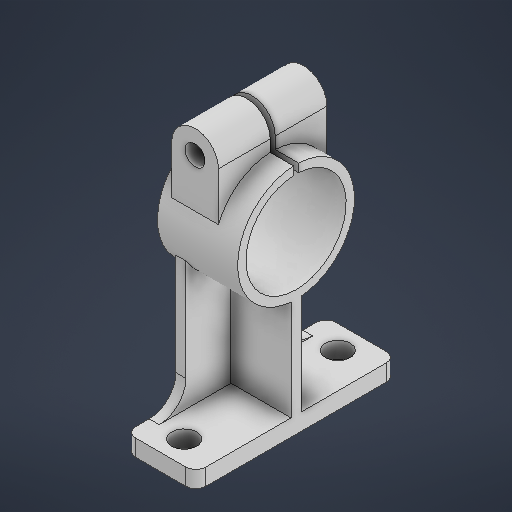
# Autodesk Inventor part: Pieza4
Saved by Autodesk Inventor 2026.1 (Build 301233020, 233B)
## iProperties
Created: 2026-02-14
Part Number: Pieza4
Material: Genérico
Document SubType Name: Modeling
Designer: UPN
Density: 1 g/cm^3
Appearance: Valor por defecto
Author: UPN
Autodesk Inventor part; units mm, degrees
note: some values were not read from the file. Chosen so that the rebuilt part matches the saved one: direction of "Hole1".
ref_plane "YZ Plane" through (0, 0, 0) normal (1, 0, 0) x (0, 1, 0)
ref_plane "XZ Plane" through (0, 0, 0) normal (0, 1, 0) x (-1, 0, 0)
sketch "Boceto1" plane through (0, 0, 0) normal (0, 1, 0) x (-1, 0, 0)
  line L0 (-15, 60) -> (15, 60)
  line L1 (21, 54) -> (21, -54)
  line L2 (15, -60) -> (-15, -60)
  line L3 (-21, -54) -> (-21, 54)
  line L4 (-21, 60) -> (21, -60) construction
  line L5 (21, 60) -> (-21, -60) construction
  arc A0 (21, 54) -> (15, 60) centre (15, 54) ccw
  arc A1 (-15, 60) -> (-21, 54) centre (-15, 54) ccw
  arc A2 (-21, -54) -> (-15, -60) centre (-15, -54) ccw
  arc A3 (15, -60) -> (21, -54) centre (15, -54) ccw
  circle A4 centre (0, 46) radius 7.5
  circle A5 centre (0, -46) radius 7.5
  point P0 (0, 0)
  dimension "d0" = 42
  dimension "d1" = 120
  dimension "d2" = 6
  dimension "d3" = 15
  dimension "d13" = 46
  dimension "d14" = 46
  constraints: 12 end point, 8 point on circle, 8 point on line, 8 tangent, 6 centre point, 4 equal radius, 2 midpoint, 2 parallel, 2 vertical alignment, 1 horizontal, 1 perpendicular
  measures "d0" distance of L4.end L5.end
  measures "d1" distance of L5.start L4.end
  measures "d2" radius of A0
  measures "d3" diameter of A4
  measures "d13" distance of A4.centre point (0, 0)
  measures "d14" distance of point (0, 0) A5.centre
extrude "Extrusión1" add sketch "Boceto1" along normal blind 10
sketch "Boceto2" plane through (-21, 0, -54) normal (-1, 0, 0) x (0, 0, 1)
  line L0 (0, 10) -> (108, 10) construction
  line L1 (24, 86.9722) -> (24, 26)
  line L2 (84, 86.9722) -> (84, 26)
  line L3 (0, 0) -> (108, 0) projected
  arc A0 (84, 26) -> (100, 10) centre (100, 26) ccw
  arc A1 (8, 10) -> (24, 26) centre (8, 26) ccw
  line L4 (92.5, 10) -> (107.5, 10) construction
  line L5 (0.5, 10) -> (15.5, 10) construction
  circle A2 centre (54, 105) radius 35
  line L6 (8, 10) -> (100, 10)
  point P0 (54, 0)
  point P1 (24, 10)
  point P2 (84, 10)
  point P3 (54, 0)
  point P4 (54, 0)
  point P5 (54, 10)
  dimension "d10" = 16
  dimension "d16" = 35
  dimension "d17" = 95
  constraints: 6 end point, 6 point on circle, 4 midpoint, 3 centre point, 3 vertical alignment, 2 point on line, 2 tangent, 2 vertical, 1 collinear, 1 equal radius, 6 other
  measures "d10" radius of A0
  measures "d16" radius of A2
  measures "d17" distance of A2.centre point (54, 10)
extrude "Extrusión2" add sketch "Boceto2" against normal blind 6 contours A2 L2 A0 L6 A1 L1
ref_plane "Plano de trabajo1" through (-18, 0, -54) normal (1, 0, 0) x (0, 0, -1)
sketch "Boceto3" plane through (-18, 0, -54) normal (1, 0, 0) x (0, 0, -1)
  arc A0 (-84, 86.9722) -> (-24, 86.9722) centre (-54, 105) ccw projected
  circle A1 centre (-54, 105) radius 35
  circle A2 centre (-54, 105) radius 30
  line L0 (-57, 10) -> (-51, 10)
  line L1 (-51, 10) -> (-51, 70.1288)
  line L2 (-51, 70.1288) -> (-57, 70.1288)
  line L3 (-57, 70.1288) -> (-57, 10)
  line L4 (-57, 10) -> (-51, 70.1288) construction
  line L5 (-51, 10) -> (-57, 70.1288) construction
  line L6 (-8, 10) -> (-100, 10) projected
  line L7 (-55.5, 105) -> (-52.5, 105)
  line L8 (-52.5, 105) -> (-52.5, 175)
  line L9 (-52.5, 175) -> (-55.5, 175)
  line L10 (-55.5, 175) -> (-55.5, 105)
  line L11 (-55.5, 105) -> (-52.5, 175) construction
  line L12 (-52.5, 105) -> (-55.5, 175) construction
  point P0 (-54, 0)
  point P1 (-54, 40.0644)
  point P2 (-54, 140)
  point P3 (-55.5, 134.9625)
  point P4 (-55.5, 139.9678)
  point P5 (-52.5, 139.9678)
  point P6 (-52.5, 134.9625)
  dimension "d23" = 39
  dimension "d20" = 30
  dimension "d21" = 6
  dimension "d22" = 3
  constraints: 24 end point, 5 midpoint, 4 parallel, 3 coincident, 3 point on circle, 2 centre point, 2 horizontal, 2 perpendicular, 2 vertical alignment, 1 collinear
  measures "d20" radius of A2
  measures "d21" distance of L0.start L0.end
  measures "d22" distance of L8.end L9.end
extrude "Extrusión3" add sketch "Boceto3" along normal up to surface (39 mm away) contours A1 L10 A2 L8 A0 L2 | L2 A0 | A0 L1 L0 L3
sketch "Boceto4" plane through (-18, 0, -54) normal (-1, 0, 0) x (0, 0, 1)
  arc A0 (24, 86.9722) -> (84, 86.9722) centre (54, 105) ccw projected
  arc A1 (84, 86.9722) -> (55.5, 139.9678) centre (54, 105) ccw projected
  line L0 (55.5, 134.9625) -> (55.5, 139.9678) projected
  arc A2 (52.5, 134.9625) -> (55.5, 134.9625) centre (54, 105) ccw projected
  line L1 (52.5, 139.9678) -> (52.5, 134.9625) projected
  arc A3 (52.5, 139.9678) -> (24, 86.9722) centre (54, 105) ccw projected
  point P0 (54, 0)
extrude "Extrusión4" add sketch "Boceto4" along normal blind 9
sketch "Sketch6" plane through (-21, 0, -54) normal (-1, 0, 0) x (0, 0, 1)
  arc A0 (52.5, 139.9678) -> (55.5, 139.9678) centre (54, 105) ccw projected
  line L0 (52.5, 139.9678) -> (52.5, 161)
  line L1 (52.5, 161) -> (21.5, 161)
  line L2 (21.5, 161) -> (21.5, 117.9904)
  line L3 (21.5, 147) -> (52.5, 147) construction
  point P0 (54, 0)
  dimension "d30" = 31
  dimension "d31" = 42
  dimension "d32" = 14
  constraints: 8 end point, 3 perpendicular, 2 point on line, 1 point on circle, 1 vertical
  measures "d30" distance of L0.end L1.end
  measures "d31" distance from line of L3 A0.centre
  measures "d32" distance between parallel lines of L1 L3
extrude "Extrusion5" add sketch "Sketch6" against normal blind 28
fillet "Fillet1" radius 14 2 edges at (7, 161, -17) (-21, 161, -17)
sketch "Sketch7" plane through (7, 117.9904, -32.5) normal (0, 0, -1) x (-1, 0, 0)
  arc A0 (28, 29.0096) -> (0, 29.0096) centre (14, 29.0096) ccw projected
  point P0 (7, -117.9904)
  constraints: 1 coincident
hole "Hole1" at (-7, 147, -32.5) direction (0, 0, 1) diameter 12 depth 31
mirror "Mirror1" about plane through (0, 0, 0) normal (0, 0, 1) of "Extrusion5", "Fillet1", "Hole1"
sketch "Sketch8" plane through (0, 0, 0) normal (0, 0, 1) x (1, 0, 0)
  line L0 (-27, 70) -> (-21, 70) projected
  line L1 (-21, 0) -> (-21, 10) projected
  line L2 (-21, 10) -> (-21, 26) projected
  line L3 (-21, 26) -> (-21, 86.9722) projected
  line L4 (-21, 86.9722) -> (-21, 86.9722) projected
  line L5 (-21, 86.9722) -> (-21, 26) projected
  line L6 (-21, 26) -> (-21, 10) projected
  line L7 (-21, 0) -> (-21, 10) projected
  line L8 (-27, 70) -> (-21, 20)
  line L9 (-27, 139.9678) -> (-27, 70) projected
  line L10 (-27, 70) -> (-27, 73)
  line L11 (-27, 73) -> (-21, 73)
  point P0 (0, 0)
  dimension "d43" = 20
  dimension "d44" = 3
  constraints: 6 end point, 3 point on line, 1 perpendicular
  measures "d43" distance of L8.end L7.start
  measures "d44" distance from line of L0.start L11
extrude "Extrusion6" add sketch "Sketch8" along normal mid plane 6
